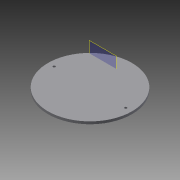
# Autodesk Inventor part: obudowa - czujnik czadu - gora
Saved by Autodesk Inventor 2014 (Build 180170000, 170)
## iProperties
Created: 2018-02-27
Part Number: obudowa - czujnik czadu - gora
Material: Generic
Document SubType Name: Modeling
Designer: HP820
Density: 1 g/cm^3
Appearance: Default
Author: HP820
Autodesk Inventor part; units mm, degrees
ref_plane "YZ Plane" through (0, 0, 0) normal (1, 0, 0) x (0, 1, 0)
ref_plane "XZ Plane" through (0, 0, 0) normal (0, 1, 0) x (-1, 0, 0)
ref_plane "XY Plane" through (0, 0, 0) normal (0, 0, 1) x (1, 0, 0)
sketch "Sketch1" plane through (0, 0, 0) normal (0, 0, 1) x (1, 0, 0)
  circle A0 centre (0, 0) radius 34 projected
  circle A1 centre (0, 0) radius 34
  arc A2 (-27.8015, 13.7141) -> (19.5355, -24.07) centre (0, 0) ccw projected
  circle A3 centre (-23.6431, 17.6424) radius 1.5 projected
  arc A4 (-27.8015, 13.7141) -> (-20.2887, 23.4387) centre (-26.2341, 20.2675) ccw projected
  arc A5 (28.3225, -12.603) -> (-20.2887, 23.4387) centre (0, 0) ccw projected
  arc A6 (28.3225, -12.603) -> (19.5355, -24.07) centre (27.5695, -21.1262) ccw projected
  circle A7 centre (23.6117, -17.6844) radius 1.5 projected
  point P0 (0, 0)
  constraints: 1 centre point, 1 coincident, 1 concentric
extrude "Extrusion1" add sketch "Sketch1" along normal blind 2 contours A0 | A4 A5 A6 A2 | A3 | A7
sketch "Sketch2" plane through (0, 0, 2) normal (0, 0, 1) x (1, 0, 0)
  circle A0 centre (0, 0) radius 34 projected
  circle A1 centre (0, 0) radius 29
  circle A2 centre (-29, 0) radius 1
  circle A3 centre (29, 0) radius 1
  dimension "d2" = 58
  dimension "d3" = 2
  dimension "d4" = 2
  constraints: 3 centre point, 2 point on circle, 1 coincident
  measures "d2" diameter of A1
  measures "d3" diameter of A2
  measures "d4" diameter of A3
extrude "Extrusion2" cut sketch "Sketch2" against normal up to next contours A1 A3 | A1 A3 | A2 A1 | A1 A2
sketch "Sketch3" plane through (0, 0, 0) normal (0, 0, -1) x (-1, 0, 0)
  circle A0 centre (-17.7645, -16.1003) radius 5 projected
  circle A1 centre (-25, 0) radius 2 projected
  circle A2 centre (0, -25) radius 2 projected
  circle A3 centre (0, 25) radius 2 projected
  circle A4 centre (25, 0) radius 2 projected
  circle A5 centre (0, 0) radius 34 projected
  circle A6 centre (-17.7645, -16.1003) radius 5 projected
  circle A7 centre (-25, 0) radius 2 projected
  circle A8 centre (0, -25) radius 2 projected
  circle A9 centre (0, 25) radius 2 projected
  circle A10 centre (25, 0) radius 2 projected
  circle A11 centre (0, 0) radius 34 projected
  circle A12 centre (-4.1956, 17.0139) radius 1.25 projected
  circle A13 centre (-4.1956, 17.0139) radius 3 projected
  circle A14 centre (14.8044, 17.0139) radius 3 projected
  circle A15 centre (-17.7645, -16.1003) radius 5 projected
  circle A16 centre (-25, 0) radius 2 projected
  circle A17 centre (0, -25) radius 2 projected
  circle A18 centre (0, 25) radius 2 projected
  circle A19 centre (25, 0) radius 2 projected
  circle A20 centre (0, 0) radius 34 projected
  circle A21 centre (-17.7645, -16.1003) radius 5 projected
  circle A22 centre (-25, 0) radius 2 projected
  circle A23 centre (0, -25) radius 2 projected
  circle A24 centre (0, 25) radius 2 projected
  circle A25 centre (25, 0) radius 2 projected
  circle A26 centre (0, 0) radius 34 projected
  circle A27 centre (14.8044, 17.0139) radius 1.25 projected
  circle A28 centre (0, -25) radius 2 projected
  circle A29 centre (0, -25) radius 4 projected
  circle A30 centre (14.8044, -16.9861) radius 3 projected
  circle A31 centre (14.8044, -16.9861) radius 1.25 projected
  circle A32 centre (-4.1956, -16.9861) radius 3 projected
  circle A33 centre (-4.1956, -16.9861) radius 1.25 projected
  circle A34 centre (-29, 0) radius 1 projected
  circle A35 centre (29, 0) radius 1 projected
  circle A36 centre (0, 0) radius 34 projected
  circle A37 centre (0, -25) radius 2 projected
  circle A38 centre (0, 25) radius 4 projected
  circle A39 centre (-25, 0) radius 4 projected
  circle A40 centre (25, 0) radius 4 projected
  arc A41 (-19.8281, -23.8295) -> (-25.6588, -17.3961) centre (0, 0) ccw projected
  arc A42 (13.2717, 27.5211) -> (-12.7645, 27.4705) centre (0.3084, -0.6906) ccw
  arc A43 (13.2717, 25.6991) -> (-12.7645, 25.8003) centre (0.1586, 1.3069) ccw
  line L0 (-12.7645, 27.4705) -> (-12.7645, 25.8003)
  line L1 (13.2717, 27.5211) -> (13.2717, 25.6991)
  constraints: 5 point on circle, 4 end point, 2 centre point, 1 parallel, 1 vertical
extrude "Extrusion3" add sketch "Sketch3" along normal blind 8 contours A43 L0 A42 L1
chamfer "Chamfer1" distance 2 angle 45 1 edges at (-0.2663, 29.0002, 0)
sketch "Sketch4" plane through (0, 0, 0) normal (0, 0, -1) x (-1, 0, 0)
  line L0 (-12.7645, 23.5139) -> (13.2717, 23.5139)
  line L1 (13.2717, 23.5139) -> (13.2717, 21.4752)
  line L2 (13.2717, 21.4752) -> (-12.7645, 21.4752)
  line L3 (-12.7645, 21.4752) -> (-12.7645, 23.5139)
  constraints: 8 end point, 2 parallel, 1 horizontal, 1 perpendicular
ref_plane "Work Plane1" through (-13.0817, 23.5139, 0) normal (0, 1, 0) x (1, 0, 0)
sketch "Sketch5" plane through (-13.0817, 23.5139, 0) normal (0, 1, 0) x (1, 0, 0)
  spline S0 degree 3 poles (13.9902, 4.2864) (13.9902, 4.1906) (13.9808, 4.0914) (13.9298, 3.8357) (13.8718, 3.6808) (13.6889, 3.361) (13.5569, 3.2131) (13.2964, 3.0152) (13.1834, 2.95) (12.8845, 2.8261) (12.6903, 2.7886) (12.3247, 2.7844) (12.1287, 2.8174) (11.7061, 2.9821) (11.4973, 3.1327) (11.2113, 3.4795) (11.1131, 3.6592) (11.0113, 3.994) (10.9902, 4.1437) (10.9902, 4.4419) (11.0154, 4.6057) (11.1112, 4.8927) (11.1738, 5.0182) (11.3265, 5.2426) (11.4138, 5.3391) (11.6377, 5.5318) (11.787, 5.6223) (12.1767, 5.7742) (12.417, 5.8034) (12.7912, 5.7625) (12.9317, 5.7272) (13.2447, 5.5974) (13.4109, 5.4852) (13.5985, 5.3001) (13.6507, 5.2402) (13.8243, 5.0041) (13.9172, 4.7969) (13.9805, 4.4843) (13.9902, 4.3837) (13.9902, 4.2864) knots 0 0 0 0 0.028257 0.028257 0.073468 0.073468 0.132242 0.132242 0.169521 0.169521 0.226024 0.226024 0.28256 0.28256 0.356364 0.356364 0.410996 0.410996 0.452121 0.452121 0.496926 0.496926 0.534877 0.534877 0.572828 0.572828 0.621682 0.621682 0.693024 0.693024 0.734722 0.734722 0.791225 0.791225 0.814453 0.814453 0.875568 0.875568 0.904243 0.904243 0.904243 0.904243 weights 1 1 1 1 1 1 1 1 1 1 1 1 1 1 1 1 1 1 1 1 1 1 1 1 1 1 1 1 1 1 1 1 1 1 1 1 1 1 1 1 projected
  point P0 (13.0817, 0)
  point P1 (13.9902, 4.2864)
extrude "Extrusion5" cut sketch "Sketch5" along normal blind 24
chamfer "Chamfer2" distance 8 angle 45 2 edges at (12.7645, 26.6354, -8) (-13.2717, 26.6101, -8)
fillet "Fillet1" radius 1 5 edges at (-0.2552, 29.0003, -8) (7.8157, 27.8275, -4.9488) (-8.3244, 27.7692, -4.9474) (11.7985, 25.1346, -0.966) (-12.3062, 25.0375, -0.9655)
body "Solid1"
